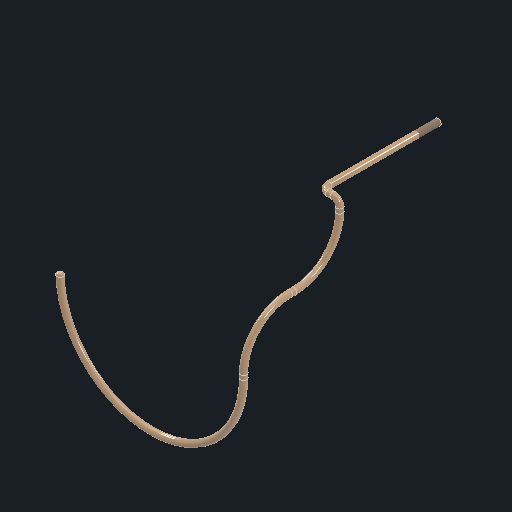
# Autodesk Inventor part: Tea Lifter Arm
Saved by Autodesk Inventor 2027.1 (Build 311270010, 270A)
## iProperties
Created: 2025-09-16
Part Number: Tea Lifter Arm
Material: Stainless Steel AISI 304
Document SubType Name: Modeling
Designer: SD
Density: 8 g/cm^3
Appearance: Brindle
Mass: 9.39372 g
Surface Area: 14.2336 cm^2
Volume: 1.05857 cm^3
Project: Automatic Tea Steeping mechanism
BOM-Mass: 0.00939
BOM-Area: 0.001
Diameter: 3.000 mm
Procurement: Fabricate - 2nd round
Build Stage: 3
Preferred Material: 304 Stainless Steel
Author: SD
Title: Tea Lifter Arm
Autodesk Inventor part; units mm, degrees
ref_plane "YZ Plane" through (0, 0, 0) normal (1, 0, 0) x (0, 1, 0)
ref_plane "XZ Plane" through (0, 0, 0) normal (0, 1, 0) x (-1, 0, 0)
ref_plane "XY Plane" through (0, 0, 0) normal (0, 0, 1) x (1, 0, 0)
sketch "Sketch1" plane through (0, 0, 0) normal (0, 0, 1) x (1, 0, 0)
  circle A0 centre (0, 0) radius 1.5
  dimension "Diameter" = 3
  constraints: 1 centre point, 1 coincident
  measures "Diameter" diameter of A0
extrude "Extrusion1" add sketch "Sketch1" along normal mid plane 50
thread "Thread1"
sketch "Sketch3" plane through (0, 0, 25) normal (0, 0, 1) x (1, 0, 0)
  circle A0 centre (0, 0) radius 1.5 projected
sketch3d "3D Sketch2"
  arc A0 (0, 0, 25) -> (3, 0, 28) centre (3, 0, 25) ccw
  line L0 (3, 0, 28) -> (5, 0, 28)
  arc A1 (5, 0, 28) -> (8, -3, 28) centre (5, -3, 28) ccw
  line L1 (8, -3, 28) -> (8, -5, 28)
  arc A2 (8, -5, 28) -> (8, -26, 49) centre (8, -5, 49) ccw
  line L2 (8, -26, 49) -> (8, -26, 51)
  arc A3 (8, -26, 51) -> (8, -47, 72) centre (8, -47, 51) ccw
  line L3 (8, -47, 72) -> (8, -49, 72)
  arc A4 (8, -49, 72) -> (-4.3015, -78.6985, 72) centre (-34, -49, 72) ccw
  arc A5 (-4.3015, -78.6985, 72) -> (-34, -91, 72) centre (-34, -49, 72) ccw
  arc A6 (-34, -91, 72) -> (-63.6985, -78.6985, 72) centre (-34, -49, 72) ccw
  arc A7 (-63.6985, -78.6985, 72) -> (-76, -49, 72) centre (-34, -49, 72) ccw
  dimension "d12" = 3
  dimension "d14" = 3
  dimension "d15" = 2
  dimension "d16" = 2
  dimension "d17" = 21
  dimension "d18" = 2
  dimension "d19" = 21
  dimension "d20" = 2
  dimension "d25" = 42
sweep "Sweep2" add profiles "Sketch3" path "3D Sketch2"
fillet "Fillet2" radius 1 1 edges at (-76, -49, 73.5)
body "Solid1"
